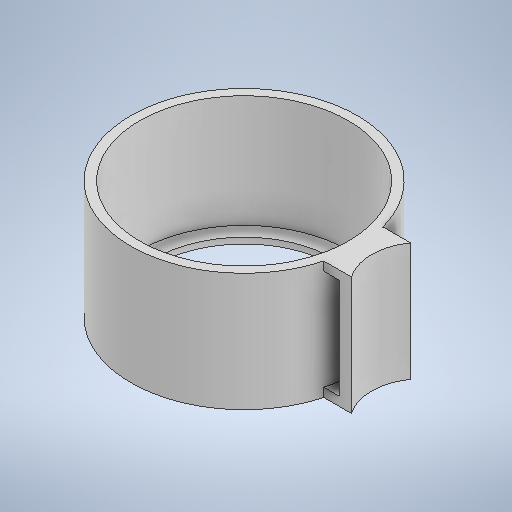
# Autodesk Inventor part: Mount
Saved by Autodesk Inventor 2025 (Build 290162010, 162A)
## iProperties
Created: 2024-07-15
Part Number: Mount
Material: Generic
Document SubType Name: Modeling
Designer: vncnt
Density: 1 g/cm^3
Appearance: Default
Author: vncnt
Autodesk Inventor part; units mm, degrees
ref_plane "YZ Plane" through (0, 0, 0) normal (1, 0, 0) x (0, 1, 0)
ref_plane "XZ Plane" through (0, 0, 0) normal (0, 1, 0) x (-1, 0, 0)
ref_plane "XY Plane" through (0, 0, 0) normal (0, 0, 1) x (1, 0, 0)
sketch "Sketch1" plane through (0, 0, 0) normal (0, 1, 0) x (-1, 0, 0)
  circle A0 centre (0, 0) radius 48.6156
  circle A1 centre (0, 0) radius 44.8056
  dimension "d0" = 97.2312
  dimension "d1" = 89.6112
  constraints: 2 centre point, 2 coincident
  measures "d0" diameter of A0
  measures "d1" diameter of A1
extrude "Extrusion1" add sketch "Sketch1" along normal blind 50.8
sketch "Sketch2" plane through (0, 0, 0) normal (0, 0, 1) x (1, 0, 0)
  line L0 (0, 0) -> (58.8549, 0)
  line L1 (58.8549, 0) -> (58.8549, 25.4)
  line L2 (0, 25.4) -> (0, 0)
  line L3 (50.4953, 3.81) -> (3.81, 3.81)
  line L4 (3.81, 3.81) -> (3.81, 21.59)
  line L5 (3.81, 21.59) -> (45.975, 21.59)
  line L6 (45.975, 21.59) -> (45.975, 3.81)
  line L7 (45.975, 21.59) -> (45.975, 25.4)
  line L8 (45.975, 3.81) -> (45.975, 0)
  line L9 (50.4953, 21.59) -> (50.4953, 3.81)
  line L10 (0, 50.8) -> (58.8549, 50.8)
  line L11 (58.8549, 50.8) -> (58.8549, 25.4)
  line L12 (50.4953, 46.99) -> (3.81, 46.99)
  line L13 (3.81, 29.21) -> (45.975, 29.21)
  line L14 (45.975, 29.21) -> (45.975, 46.99)
  line L15 (45.975, 29.21) -> (45.975, 25.4)
  line L16 (45.975, 46.99) -> (45.975, 50.8)
  line L17 (50.4953, 29.21) -> (50.4953, 46.99)
  line L18 (50.4953, 29.21) -> (50.4953, 21.59)
  line L19 (45.975, 25.4) -> (0, 25.4)
  constraints: 40 end point, 6 point on line, 4 perpendicular, 3 parallel, 1 horizontal, 1 vertical
extrude "Extrusion2" add sketch "Sketch2" along normal mid plane 25.4 contours L8 L3 L9 L18 L17 L12 L16 L10 L11 L1 L0
sketch "Sketch3" plane through (0, 0, 0) normal (0, -1, 0) x (1, 0, 0)
  circle A0 centre (0, 0) radius 44.8056
  circle A1 centre (0, 0) radius 38.608
  dimension "d7" = 77.216
  constraints: 2 centre point, 2 coincident
  measures "d7" diameter of A1
extrude "Extrusion3" add sketch "Sketch3" against normal blind 2.54
sketch "Sketch4" plane through (0, 50.8, 0) normal (0, 1, 0) x (1, 0, 0)
  line L0 (58.8549, -12.7) -> (58.8549, 12.7)
  arc A0 (58.8549, 12.7) -> (58.8549, -12.7) centre (76.984, 0) ccw
  point P0 (0, 0)
  constraints: 2 end point, 2 point on circle, 1 centre point
sketch "Sketch5" plane through (46.9275, 3.81, 12.7) normal (0, 1, 0) x (1, 0, 0)
  arc A0 (6.5029, 25.4) -> (6.6061, 0) centre (32.0653, 12.8036) ccw
  line L0 (6.5029, 25.4) -> (1.7839, 25.4)
  line L1 (0, 25.4) -> (3.5678, 25.4) projected
  line L2 (1.7839, 25.4) -> (2.3688, 0)
  line L3 (3.5678, 0) -> (0, 0) projected
  line L4 (6.6061, 0) -> (2.3688, 0)
  point P0 (-46.9275, 12.7)
  point P1 (6.5578, 0.0965)
  constraints: 6 end point, 3 point on circle, 1 centre point, 1 collinear, 1 midpoint, 1 point on line
extrude "Extrusion4" cut sketch "Sketch5" along normal up to surface (43.18 mm away)
extrude "Extrusion5" cut sketch "Sketch4" against normal up to surface (50.8 mm away)
body "Solid1"
